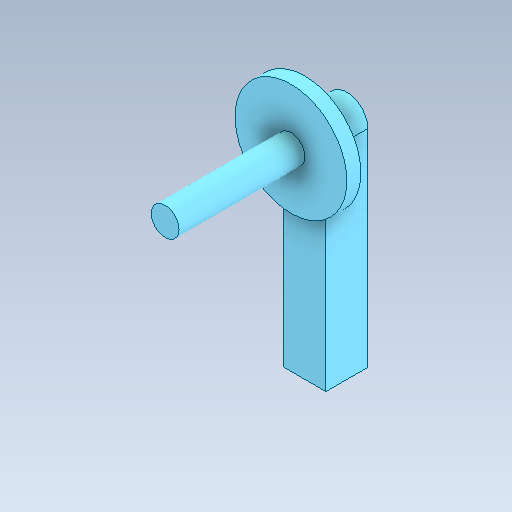
# Autodesk Inventor part: outerGear_2
Saved by Autodesk Inventor 2020.1 (Build 241239000, 239)
## iProperties
Created: 2020-01-18
Part Number: outerGear_2
Material: Generic
Document SubType Name: Modeling
Designer: Ali
Density: 1 g/cm^3
Appearance: Default
Author: Ali
Autodesk Inventor part; units mm, degrees
ref_plane "YZ Plane" through (0, 0, 0) normal (1, 0, 0) x (0, 1, 0)
ref_plane "XZ Plane" through (0, 0, 0) normal (0, 1, 0) x (-1, 0, 0)
ref_plane "XY Plane" through (0, 0, 0) normal (0, 0, 1) x (1, 0, 0)
sketch "Sketch1" plane through (0, 0, 0) normal (0, 0, 1) x (1, 0, 0)
  circle A0 centre (0, 0) radius 25.4
  dimension "d0" = 50.8
  constraints: 1 centre point, 1 coincident
  measures "d0" diameter of A0
extrude "Extrusion1" add sketch "Sketch1" along normal blind 6.35
sketch "Sketch2" plane through (0, 0, 6.35) normal (0, 0, 1) x (1, 0, 0)
  circle A0 centre (0, 0) radius 6.35
  dimension "d3" = 12.7
  constraints: 1 centre point, 1 coincident
  measures "d3" diameter of A0
extrude "Extrusion2" add sketch "Sketch2" along normal blind 57.15
sketch "Sketch3" plane through (0, 0, 0) normal (0, 0, -1) x (-1, 0, 0)
  circle A0 centre (0, 0) radius 6.35 projected
  circle A1 centre (0, 0) radius 9.525
  dimension "d6" = 19.05
  constraints: 1 centre point, 1 coincident
  measures "d6" diameter of A1
extrude "Extrusion3" add sketch "Sketch3" along normal blind 19.05
sketch "Sketch4" plane through (0, 0, -19.05) normal (0, 0, -1) x (-1, 0, 0)
  circle A0 centre (0, 0) radius 9.525 projected
  circle A1 centre (0, 0) radius 9.525 construction
  line L0 (-9.525, 0) -> (9.525, 0) construction
  line L1 (-9.525, 0) -> (9.525, 0)
  line L2 (9.525, 0) -> (9.525, -93.9249)
  line L3 (9.525, -93.9249) -> (-9.525, -93.9249)
  line L4 (-9.525, -93.9249) -> (-9.525, 0)
  dimension "d9" = 19.05
  dimension "d10" = 93.9249
  constraints: 10 end point, 2 horizontal, 2 parallel, 2 point on circle, 1 perpendicular
  measures "d9" distance between parallel lines of L4 L2
  measures "d10" distance of L1.end L2.end
extrude "Extrusion4" add sketch "Sketch4" against normal blind 19.05 contours L2 L3 L4 A0
extrude "Extrusion6" add sketch "Sketch3" along normal blind 19.05 contours A0
equation "\"d0\" = OG_gearDiameter"
equation "\"d1\" = OG_gearThickness"
equation "\"d3\" = OG_shaftDiameter"
equation "\"d4\" = OG_shaftLength"
equation "\"d6\" = LE_baseDiameter"
equation "\"d7\" = LE_thickness"
equation "\"d9\" = LE_thickness"
equation "\"d10\" = LE_maxLength"
equation "\"d11\" = LE_thickness"
equation "\"d15\" = LE_thickness + LE_offsetAboveOuterGear"
equation "\"Wheel_Related_W_\" = 0"
equation "\"W_innerDiameter\" = 254"
equation "\"W_innerDepth\" = 50.8"
equation "\"W_wallThickness\" = 6.35"
equation "\"W_holesClearance\" = 0.254"
equation "\"W_outerGearHoleDiameter\" = 13.208"
equation "\"W_innerGearHoleDiameter\" = 38.608"
equation "\"TempSpotReserved7\" = 0"
equation "\"TempSpotReserved8\" = 0"
equation "\"TempSpotReserved9\" = 0"
equation "\"TempSpotReserved10\" = 0"
equation "\"TempSpotReserved11\" = 0"
equation "\"TempSpotReserved12\" = 0"
equation "\"TempSpotReserved13\" = 0"
equation "\"TempSpotReserved14\" = 0"
equation "\"TempSpotReserved15\" = 0"
equation "\"TempSpotReserved16\" = 0"
equation "\"TempSpotReserved17\" = 0"
equation "\"TempSpotReserved18\" = 0"
equation "\"TempSpotReserved19\" = 0"
equation "\"TempSpotReserved20\" = 0"
equation "\"Inner_Gear_Related_IG_\" = 0"
equation "\"IG_shaftDiameter\" = 25.4"
equation "\"IG_gearDiameter\" = 127"
equation "\"IG_shaftLength\" = 127"
equation "\"IG_gearThickness\" = 6.35"
equation "\"TempSpotReserved25\" = 0"
equation "\"TempSpotReserved26\" = 0"
equation "\"TempSpotReserved27\" = 0"
equation "\"TempSpotReserved28\" = 0"
equation "\"TempSpotReserved29\" = 0"
equation "\"TempSpotReserved30\" = 0"
equation "\"TempSpotReserved31\" = 0"
equation "\"TempSpotReserved32\" = 0"
equation "\"TempSpotReserved33\" = 0"
equation "\"TempSpotReserved34\" = 0"
equation "\"TempSpotReserved35\" = 0"
equation "\"TempSpotReserved36\" = 0"
equation "\"TempSpotReserved37\" = 0"
equation "\"TempSpotReserved38\" = 0"
equation "\"TempSpotReserved39\" = 0"
equation "\"TempSpotReserved40\" = 0"
equation "\"Outer_Gear_Related_OG_\" = 0"
equation "\"OG_distanceFromCenter\" = 88.9"
equation "\"OG_shaftDiameter\" = 12.7"
equation "\"OG_gearDiameter\" = 50.8"
equation "\"OG_shaftLength\" = 57.15"
equation "\"OG_gearThickness\" = 6.35"
equation "\"TempSpotReserved47\" = 0"
equation "\"TempSpotReserved48\" = 0"
equation "\"TempSpotReserved49\" = 0"
equation "\"TempSpotReserved50\" = 0"
equation "\"TempSpotReserved51\" = 0"
equation "\"TempSpotReserved52\" = 0"
equation "\"TempSpotReserved53\" = 0"
equation "\"TempSpotReserved54\" = 0"
equation "\"TempSpotReserved55\" = 0"
equation "\"TempSpotReserved56\" = 0"
equation "\"TempSpotReserved57\" = 0"
equation "\"TempSpotReserved58\" = 0"
equation "\"TempSpotReserved59\" = 0"
equation "\"TempSpotReserved60\" = 0"
equation "\"Leg_Extensions_Related_LE_\" = 0"
equation "\"LE_baseDiameter\" = 19.05"
equation "\"LE_maxLength\" = 93.92488"
equation "\"LE_thickness\" = 19.05"
equation "\"IG_ratioToOuterGear\" = 2.5"
equation "\"B_bearingThickness\" = 6.35"
equation "\"TempSpotReserved43\" = 0"
equation "\"TempSpotReserved45\" = 0"
equation "\"Thisisatest\" = 25.4"
equation "\"TempSpotReserved46\" = 0"
equation "\"TempSpotReserved44\" = 0"
equation "\"LE_offsetAboveOuterGear\" = 0"
equation "\"Bearing_Related_B_\" = 0"
equation "\"TempSpotReserved42\" = 0"
body "Solid1"
